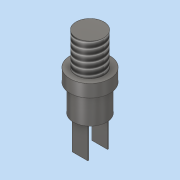
# Autodesk Inventor part: PushSwitchBody
Saved by Autodesk Inventor 2017 (Build 210142000, 142)
## iProperties
Created: 2016-12-03
Part Number: PushSwitchBody
Material: Stainless Steel
Document SubType Name: Modeling
Designer: techn
Density: 8 g/cm^3
Appearance: Semi-Polished
Author: techn
Autodesk Inventor part; units mm, degrees
ref_plane "YZ Plane" through (0, 0, 0) normal (1, 0, 0) x (0, 1, 0)
ref_plane "XZ Plane" through (0, 0, 0) normal (0, 1, 0) x (-1, 0, 0)
ref_plane "XY Plane" through (0, 0, 0) normal (0, 0, 1) x (1, 0, 0)
sketch "Sketch1" plane through (0, 0, 0) normal (0, 0, 1) x (1, 0, 0)
  line L0 (0, 0) -> (4.0132, 0)
  line L1 (4.0132, 0) -> (4.0132, 6.477)
  line L2 (4.0132, 6.477) -> (0, 6.477)
  line L3 (0, 6.477) -> (0, 0)
  line L4 (0, 6.477) -> (4.826, 6.477)
  line L5 (4.826, 6.477) -> (4.826, 9.525)
  line L6 (4.826, 9.525) -> (0, 9.525)
  line L7 (0, 9.525) -> (0, 6.477)
  line L8 (0, 9.525) -> (3.3655, 9.525)
  line L9 (3.3655, 9.525) -> (3.3655, 17.399)
  line L10 (3.3655, 17.399) -> (0, 17.399)
  line L11 (0, 17.399) -> (0, 9.525)
  dimension "d0" = 4.0132
  dimension "d1" = 6.477
  dimension "d2" = 4.826
  dimension "d3" = 3.048
  dimension "d4" = 3.3655
  dimension "d5" = 7.874
  constraints: 24 end point, 6 parallel, 3 horizontal, 3 perpendicular
  measures "d0" distance of L2.end L1.end
  measures "d1" distance of L1.end L0.end
  measures "d2" distance of L6.end L5.end
  measures "d3" distance of L4.end L5.end
  measures "d4" distance of L10.end L9.end
  measures "d5" distance of L9.end L8.end
revolve "Revolution1" add sketch "Sketch1" angle 360 about axis through (0, 17.399, 0) along (0, -1, 0)
thread "Thread1" size "5/16-18 UNC" class "2A" standard "ANSI Unified Screw Threads" full length
sketch "Sketch2" plane through (0, 0, 0) normal (0, -1, 0) x (1, 0, 0)
  line L0 (1.9693, -2.286) -> (-1.8407, -2.286)
  line L1 (-1.8407, -2.286) -> (-1.8407, -2.4989)
  line L2 (-1.8407, -2.4989) -> (1.9693, -2.4989)
  line L3 (1.9693, -2.4989) -> (1.9693, -2.286)
  line L4 (3.0926, 0) -> (-3.1405, 0)
  line L5 (1.9693, 2.286) -> (-1.8407, 2.286)
  line L6 (-1.8407, 2.286) -> (-1.8407, 2.4989)
  line L7 (-1.8407, 2.4989) -> (1.9693, 2.4989)
  line L8 (1.9693, 2.4989) -> (1.9693, 2.286)
  point P0 (0, 0)
  dimension "d9" = 3.81
  dimension "d10" = 2.286
  constraints: 18 end point, 4 symmetric about line, 2 horizontal, 2 parallel, 1 perpendicular, 1 point on line
  measures "d9" distance of L2.end L1.end
  measures "d10" distance between parallel lines of L0 L4
extrude "Extrusion1" add sketch "Sketch2" along normal blind 7.874
body "Solid1"
